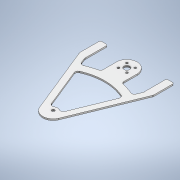
# Autodesk Inventor part: frame_rotor
Saved by Autodesk Inventor 2021 (Build 250183000, 183)
## iProperties
Created: 2022-10-22
Part Number: frame_rotor
Material: Aluminum 6061
Document SubType Name: Modeling
Designer: ermoz
Density: 2.7 g/cm^3
Appearance: Aluminum - Flat
Author: ermoz
Autodesk Inventor part; units mm, degrees
ref_plane "YZ Plane" through (0, 0, 0) normal (1, 0, 0) x (0, 1, 0)
ref_plane "XZ Plane" through (0, 0, 0) normal (0, 1, 0) x (-1, 0, 0)
ref_plane "XY Plane" through (0, 0, 0) normal (0, 0, 1) x (1, 0, 0)
sketch "Sketch1" plane through (0, 0, 0) normal (0, 1, 0) x (-1, 0, 0)
  line L0 (0, 0) -> (5.6922, -5.6922)
  line L1 (0, 0) -> (8.05, 0) construction
  circle A0 centre (5.6922, -5.6922) radius 1.5
  circle A1 centre (5.6922, 5.6922) radius 1.5
  circle A2 centre (-5.6922, 5.6922) radius 1.5
  circle A3 centre (-5.6922, -5.6922) radius 1.5
  circle A4 centre (0, 100) radius 14
  circle A5 centre (0, 100) radius 2
  line L2 (-50, -14) -> (50, -14)
  line L3 (50, -14) -> (50, 14)
  line L4 (50, 14) -> (-50, 14)
  line L5 (-50, 14) -> (-50, -14)
  line L6 (-50, -14) -> (50, 14) construction
  line L7 (50, -14) -> (-50, 14) construction
  circle A6 centre (0, 0) radius 14
  line L8 (-50, 14) -> (-12.9729, 105.2633)
  line L9 (12.9729, 105.2633) -> (50, 14)
  line L10 (10.3153, 90.5346) -> (41.3666, 14)
  line L11 (-10.3153, 90.5346) -> (-41.3666, 14)
  line L12 (0, 86) -> (0, 14)
  circle A7 centre (0, 100) radius 6
  line L13 (-10.3153, 90.5346) -> (-5.5598, 102.2557)
  line L14 (10.3153, 90.5346) -> (5.5598, 102.2557)
  line L15 (-40, 14) -> (-40, -14)
  line L16 (40, 13) -> (40, -14)
  circle A8 centre (0, 0) radius 4
  circle A9 centre (0, 100) radius 70
  circle A10 centre (0, 100) radius 80
  line L17 (-40, 14) -> (-40, 30.718)
  line L18 (-14, 0) -> (-14, 21.2345)
  line L19 (14, 0) -> (14, 21.2345)
  line L20 (40, 13) -> (40, 30.718)
  line L21 (41.3666, 14) -> (40, 12.0487)
  line L22 (-41.3666, 14) -> (-40, 17.3685)
  point P0 (4, 86.5836)
  point P1 (2.5, 14)
  point P2 (-4, 86.5836)
  point P3 (4, 95.5279)
  point P4 (-4, 95.5279)
  point P5 (4.6667, 30.1557)
  point P6 (-4.6667, 30.1557)
  point P7 (31.7797, 37.6297)
  point P8 (-31.7797, 37.6297)
  point P9 (-42.585, 32.2762)
  point P10 (-14, 14)
  point P11 (14, 14)
  point P12 (42.585, 32.2762)
  point P13 (40, 14)
  point P14 (40, 38.6477)
  point P15 (0, 14)
  point P16 (-40, 38.6477)
  point P17 (-40, 17.3685)
  point P18 (-35.5513, 28.3334)
  point P19 (40, 17.3685)
  point P20 (35.5513, 28.3334)
  dimension "d7" = 28
  dimension "d0" = 8.05
  dimension "d1" = 45
  dimension "d2" = 3
  dimension "d5" = 360
  dimension "d9" = 4
  dimension "d10" = 100
  dimension "d11" = 28
  dimension "d12" = 28
  dimension "d13" = 8
  dimension "d14" = 8
  dimension "d20" = 10
  dimension "d22" = 10
  dimension "d24" = 8
  dimension "d26" = 140
  dimension "d29" = 10
  dimension "d30" = 100
  constraints: 46 end point, 12 point on circle, 10 centre point, 9 point on line, 6 coincident, 6 parallel, 5 tangent, 3 midpoint, 3 perpendicular, 2 horizontal, 2 vertical, 1 collinear, 1 equal length, 20 other
  measures "d0" distance of L0.start L0.end
  measures "d1" angle of L0 L1
  measures "d2" diameter of A0
  measures "d9" diameter of A5
  measures "d10" distance of L2.start L2.end
  measures "d11" distance between parallel lines of L2 L4
  measures "d12" diameter of A6
  measures "d13" distance between parallel lines of L10 L9
  measures "d14" distance between parallel lines of L8 L11
  measures "d20" distance between parallel lines of L3 L16
  measures "d22" distance between parallel lines of L5 L15
  measures "d24" diameter of A8
  measures "d26" diameter of A9
  measures "d29" radial gap between concentric circles of A9 A10
  measures "d30" distance of L0.start point (0, 100)
extrude "Extrusion1" add sketch "Sketch1" along normal blind 2 contours A4 L14 A7 L13 | A4 L9 A9 L10 | A4 L11 A9 L8 | L9 A10 L10 A9 | L10 A10 L12 A9 | A7 | A9 L11 A10 L8 | L9 L4 L10 L20 A10 | L12 A10 L11 A9 | A10 L20 L10 | A10 L17 L11 L4 L8 | L3 L2 L16 L21 L4 | A10 L19 L4 L12 | L12 L4 L18 A10 | L10 L4 L20 | L11 L17 A10 | L4 L15 L2 L5 | L21 L16 L20 L4 | A6 L18 L4 | L4 L19 A6 | A6 | L17 L4 L11 picked at (9.3983, 95.3801)
fillet "Fillet1" radius 4 6 edges at (5.5598, 1, 102.2557) (-5.5598, 1, 102.2557) (50, 1, 14) (-50, 1, 14) (-31.7797, 1, 37.6297) (31.7797, 1, 37.6297)
fillet "Fillet2" radius 4 6 edges at (14, 1, 21.2345) (-14, 1, 21.2345) (35.5513, 1, 28.3334) (40, 1, 17.3685) (-35.5513, 1, 28.3334) (-40, 1, 17.3685)
fillet "Fillet3" radius 2 4 edges at (-40, 1, -14) (50, 1, -14) (40, 1, -14) (-50, 1, -14)
equation "\"d14\" = d13"
equation "\"d20\" = d22"
body "Solid1"
